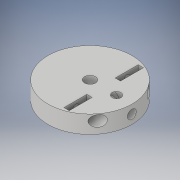
# Autodesk Inventor part: table
Saved by Autodesk Inventor 2018 (Build 220112000, 112)
## iProperties
Created: 2018-07-02
Part Number: table
Material: Generic
Document SubType Name: Modeling
Designer: Cole Tucker
Density: 1 g/cm^3
Appearance: Default
Author: Cole Tucker
Autodesk Inventor part; units mm, degrees
ref_plane "YZ Plane" through (0, 0, 0) normal (1, 0, 0) x (0, 1, 0)
ref_plane "XZ Plane" through (0, 0, 0) normal (0, 1, 0) x (-1, 0, 0)
ref_plane "XY Plane" through (0, 0, 0) normal (0, 0, 1) x (1, 0, 0)
sketch "Sketch1" plane through (0, 0, 0) normal (0, 1, 0) x (-1, 0, 0)
  circle A0 centre (0, 0) radius 24.13
  dimension "d0" = 48.26
  constraints: 1 centre point, 1 coincident
  measures "d0" diameter of A0
extrude "Extrusion1" add sketch "Sketch1" along normal blind 10.16
sketch "Sketch2" plane through (0, 10.16, 0) normal (0, 1, 0) x (1, 0, 0)
  line L0 (0, 0) -> (12.7, 0)
  line L1 (6.35, 0) -> (6.35, -21.336)
  line L2 (6.35, -21.336) -> (9.398, -21.336)
  line L3 (9.398, -21.336) -> (9.398, -8.128)
  line L4 (9.398, -8.128) -> (6.35, -8.128)
  line L5 (6.35, 0) -> (6.35, 21.336)
  line L6 (6.35, 21.336) -> (9.398, 21.336)
  line L7 (9.398, 21.336) -> (9.398, 8.128)
  line L8 (9.398, 8.128) -> (6.35, 8.128)
  dimension "d3" = 12.7
  dimension "d4" = 21.336
  dimension "d6" = 3.048
  dimension "d7" = 13.208
  constraints: 18 end point, 4 symmetric about line, 2 horizontal, 2 perpendicular, 2 point on line, 1 midpoint, 1 vertical
  measures "d3" distance of L0.start L0.end
  measures "d4" distance of L1.start L1.end
  measures "d6" distance of L1.end L2.end
  measures "d7" distance of L2.end L3.end
extrude "Extrusion2" cut sketch "Sketch2" against normal blind 8.89
sketch "Sketch3" plane through (6.35, 10.16, 21.336) normal (1, 0, 0) x (0, 0, -1)
  line L0 (13.208, 0) -> (0, 0) projected
  line L1 (0, -8.89) -> (13.208, -8.89) projected
  line L2 (29.972, 0) -> (43.18, 0) projected
  line L3 (29.972, -8.89) -> (43.18, -8.89) projected
  circle A0 centre (6.858, -3.556) radius 1.905
  circle A1 centre (36.322, -3.556) radius 1.905
  line L4 (45.466, 0) -> (-2.794, 0) projected
  line L5 (43.18, 0) -> (43.18, -8.89) projected
  line L6 (43.18, 0) -> (36.322, 0)
  line L7 (36.322, 0) -> (36.322, -3.556)
  line L8 (0, 0) -> (6.858, 0)
  line L9 (6.858, 0) -> (6.858, -3.556)
  point P0 (21.336, -10.16)
  dimension "d17" = 3.81
  dimension "d18" = 3.81
  dimension "d42" = 6.858
  dimension "d43" = 3.556
  dimension "d44" = 6.858
  dimension "d45" = 3.556
  constraints: 8 end point, 2 centre point, 2 perpendicular, 2 point on line
  measures "d17" diameter of A0
  measures "d18" diameter of A1
  measures "d42" distance of L2.end L6.end
  measures "d43" distance of L6.end L7.end
  measures "d44" distance of L0.end L8.end
  measures "d45" distance of L8.end L9.end
extrude "Extrusion3" cut sketch "Sketch3" against normal blind 12.7
sketch "Sketch4" plane through (6.35, 10.16, 21.336) normal (1, 0, 0) x (0, 0, -1)
  circle A0 centre (6.858, -3.556) radius 1.905 projected
  circle A1 centre (6.858, -3.556) radius 3.175
  circle A2 centre (36.322, -3.556) radius 1.905 projected
  circle A3 centre (36.322, -3.556) radius 3.175
  point P0 (21.336, -10.16)
  dimension "d21" = 6.35
  dimension "d22" = 6.35
  constraints: 2 centre point, 2 coincident
  measures "d21" diameter of A1
  measures "d22" diameter of A3
extrude "Extrusion4" cut sketch "Sketch4" along normal blind 25.4 contours A0 | A1 | A2 | A3
sketch "Sketch7" plane through (0, 10.16, 0) normal (0, 1, 0) x (1, 0, 0)
  circle A0 centre (0, 0) radius 3.175
  dimension "d33" = 6.35
  constraints: 1 centre point, 1 coincident
  measures "d33" diameter of A0
extrude "Extrusion6" cut sketch "Sketch7" against normal blind 12.7
fillet "Fillet2" radius 3.175 4 edges at (7.874, 1.27, 21.336) (7.874, 1.27, -8.128) (7.874, 1.27, -21.336) (7.874, 1.27, 8.128)
ref_plane "Work Plane3" through (-0.635, 10.16, 0) normal (-1, 0, 0) x (0, -1, 0)
ref_plane "Work Plane2" through (-3.175, 10.16, 0) normal (-1, 0, 0) x (0, -1, 0)
sketch "Sketch9" plane through (-0.635, 10.16, 0) normal (-1, 0, 0) x (0, -1, 0)
  line L0 (0, 24.13) -> (0, -24.13) projected
  line L1 (0, 0) -> (5.08, 0)
  circle A0 centre (5.08, 0) radius 2.54
  point P0 (10.16, 0)
  dimension "d63" = 5.08
  dimension "d64" = 5.08
  constraints: 2 end point, 1 centre point, 1 coincident, 1 horizontal, 1 midpoint
  measures "d63" distance of L1.start L1.end
  measures "d64" diameter of A0
extrude "Extrusion8" cut sketch "Sketch9" against normal blind 50.8
fillet "Fillet4" radius 3.175 2 edges at (1.905, 5.0808, 2.54) (1.905, 5.0792, -2.54)
sketch "Sketch10" plane through (0, 10.16, 0) normal (0, 1, 0) x (1, 0, 0)
  line L0 (0, 0) -> (15.24, 0)
  circle A0 centre (15.24, 0) radius 2.54
  dimension "d68" = 15.24
  dimension "d69" = 5.08
  constraints: 2 end point, 1 centre point, 1 coincident, 1 horizontal
  measures "d68" distance of L0.start L0.end
  measures "d69" diameter of A0
extrude "Extrusion9" cut sketch "Sketch10" against normal blind 5.08
fillet "Fillet5" radius 3.175 4 edges at (13.4439, 6.8761, 1.7961) (13.4439, 6.8761, -1.7961) (17.0361, 6.8761, 1.7961) (17.0361, 6.8761, -1.7961)
body "Solid1"
